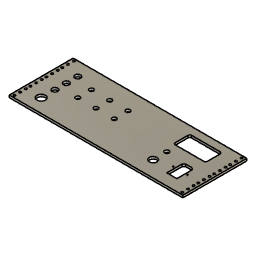
front_panel_3 v4 (Autodesk Fusion 360 design; units mm, degrees)
Autodesk Fusion 360 part; units mm, degrees
sketch "Sketch1" plane through (0, 0, 0) normal (0, 0, 1) x (1, 0, 0)
  line L0 (0, 0) -> (482.6, 0)
  line L1 (482.6, 0) -> (482.6, 177.8)
  line L2 (482.6, 177.8) -> (0, 177.8)
  line L3 (0, 177.8) -> (0, 0)
  dimension "d1" = 482.6
  dimension "d2" = 177.8
  constraint horizontal L0
  constraint vertical L1
  constraint horizontal L2
  constraint vertical L3
  constraint coincident L0.start L3.end
  measures "d1" distance of L0.start L0.end
  measures "d2" distance of L0.start L2.end
extrude "Extrude1" add sketch "Sketch1" along normal blind 6.35
sketch "Sketch2" plane through (0, 0, 6.35) normal (0, 0, 1) x (-1, 0, 0)
  line L0 (0, -177.8) -> (0, 0)
  line L1 (0, 0) -> (-482.6, 0)
  line L2 (-482.6, 0) -> (-482.6, -177.8)
  line L3 (-482.6, -177.8) -> (0, -177.8)
  circle A0 centre (-7.9375, -6.35) radius 3
  circle A1 centre (-7.9375, -22.225) radius 3
  circle A2 centre (-7.9375, -38.1) radius 3
  line L4 (-482.6, -88.9) -> (0, -88.9)
  line L5 (-241.3, -177.8) -> (-241.3, 0)
  line L6 (0, -44.45) -> (-482.6, -44.45)
  circle A3 centre (-7.9375, -50.8) radius 3
  circle A4 centre (-7.9375, -66.675) radius 3
  circle A5 centre (-7.9375, -82.55) radius 3
  circle A6 centre (-7.9375, -171.45) radius 3
  circle A7 centre (-7.9375, -155.575) radius 3
  circle A8 centre (-7.9375, -127) radius 3
  circle A9 centre (-7.9375, -111.125) radius 3
  circle A10 centre (-7.9375, -95.25) radius 3
  circle A11 centre (-7.9375, -139.7) radius 3
  circle A12 centre (-474.6625, -171.45) radius 3
  circle A13 centre (-474.6625, -155.575) radius 3
  circle A14 centre (-474.6625, -139.7) radius 3
  circle A15 centre (-474.6625, -127) radius 3
  circle A16 centre (-474.6625, -111.125) radius 3
  circle A17 centre (-474.6625, -95.25) radius 3
  circle A18 centre (-474.6625, -82.55) radius 3
  circle A19 centre (-474.6625, -66.675) radius 3
  circle A20 centre (-474.6625, -50.8) radius 3
  circle A21 centre (-474.6625, -38.1) radius 3
  circle A22 centre (-474.6625, -22.225) radius 3
  circle A23 centre (-474.6625, -6.35) radius 3
  point P0 (-7.3025, -3.751)
  dimension "d5" = 6
  dimension "d6" = 6
  dimension "d7" = 6
  dimension "d8" = 15.875
  dimension "d9" = 15.875
  dimension "d10" = 7.9375
  dimension "d11" = 6.35
  dimension "d12" = 44.45
  dimension "d15" = 31.75
  constraint midpoint L2 L4.start
  constraint midpoint L0 L4.end
  constraint midpoint L3 L5.start
  constraint midpoint L1 L5.end
  constraint coincident L0 L6.start
  constraint coincident L2 L6.end
  constraint perpendicular L2 L6
  constraint symmetric A0 L6 A5
  constraint symmetric A1 L6 A4
  constraint symmetric A2 L6 A3
  constraint symmetric A0 L4 A6
  constraint symmetric A1 L4 A7
  constraint symmetric A2 L4 A11
  constraint symmetric L4 A3 A8
  constraint symmetric L4 A4 A9
  constraint symmetric L4 A5 A10
  constraint symmetric A0 L5 A23
  constraint symmetric A1 L5 A22
  constraint symmetric A2 L5 A21
  constraint symmetric L5 A3 A20
  constraint symmetric L5 A4 A19
  constraint symmetric L5 A5 A18
  constraint symmetric L5 A6 A12
  constraint symmetric L5 A7 A13
  constraint symmetric L5 A8 A15
  constraint symmetric L5 A9 A16
  constraint symmetric L5 A10 A17
  constraint symmetric L5 A11 A14
  measures "d5" diameter of A0
  measures "d6" diameter of A2
  measures "d7" diameter of A1
  measures "d8" distance of A0.centre A1.centre
  measures "d9" distance of A2.centre A1.centre
  measures "d10" distance of L0 A0.centre
  measures "d11" distance of L1 A0.centre
  measures "d12" distance of L1 L6
  measures "d15" distance of A2.centre A0.centre
extrude "Extrude2" cut sketch "Sketch2" against normal blind 6.35 contours A0 | A1 | A2 | A3 | A4 | A5 | A6 | A7 | A8 | A9 | A10 | A11 | A12 | A13 | A14 | A15 | A16 | A17 | A18 | A19 | A20 | A21 | A22 | A23
sketch "Sketch3" plane through (0, 0, 6.35) normal (0, 0, 1) x (-1, 0, 0)
  circle A0 centre (-474.6625, -38.1) radius 3
  circle A1 centre (-474.6625, -171.45) radius 3
  circle A2 centre (-474.6625, -139.7) radius 3
  circle A3 centre (-7.9375, -38.1) radius 3
  circle A4 centre (-7.9375, -95.25) radius 3
  circle A5 centre (-7.9375, -155.575) radius 3
  circle A6 centre (-7.9375, -139.7) radius 3
  circle A7 centre (-7.9375, -82.55) radius 3
  circle A8 centre (-7.9375, -22.225) radius 3
  circle A9 centre (-474.6625, -127) radius 3
  circle A10 centre (-474.6625, -82.55) radius 3
  circle A11 centre (-474.6625, -22.225) radius 3
  circle A12 centre (-474.6625, -50.8) radius 3
  circle A13 centre (-474.6625, -95.25) radius 3
  circle A14 centre (-474.6625, -155.575) radius 3
  circle A15 centre (-7.9375, -50.8) radius 3
  circle A16 centre (-7.9375, -111.125) radius 3
  circle A17 centre (-7.9375, -171.45) radius 3
  circle A18 centre (-7.9375, -127) radius 3
  circle A19 centre (-7.9375, -66.675) radius 3
  circle A20 centre (-7.9375, -6.35) radius 3
  circle A21 centre (-474.6625, -111.125) radius 3
  circle A22 centre (-474.6625, -66.675) radius 3
  circle A23 centre (-474.6625, -6.35) radius 3
  line L0 (0, -177.8) -> (0, 0)
  line L1 (0, 0) -> (-482.6, 0)
  line L2 (-482.6, 0) -> (-482.6, -177.8)
  line L3 (-482.6, -177.8) -> (0, -177.8)
  circle A24 centre (-50.8, -38.1) radius 11.9062
  dimension "d16" = 23.8125
  dimension "d17" = 38.1
  dimension "d18" = 50.8
  measures "d16" diameter of A24
  measures "d17" distance of L1 A24.centre
  measures "d18" distance of L0 A24.centre
extrude "Extrude3" cut sketch "Sketch3" against normal blind 6.35 contours A24
sketch "Sketch5" plane through (0, 0, 6.35) normal (0, 0, 1) x (-1, 0, 0)
  circle A0 centre (-50.8, -38.1) radius 11.9062
  circle A1 centre (-474.6625, -38.1) radius 3
  circle A2 centre (-474.6625, -171.45) radius 3
  circle A3 centre (-474.6625, -139.7) radius 3
  circle A4 centre (-7.9375, -38.1) radius 3
  circle A5 centre (-7.9375, -95.25) radius 3
  circle A6 centre (-7.9375, -155.575) radius 3
  circle A7 centre (-7.9375, -139.7) radius 3
  circle A8 centre (-7.9375, -82.55) radius 3
  circle A9 centre (-7.9375, -22.225) radius 3
  circle A10 centre (-474.6625, -127) radius 3
  circle A11 centre (-474.6625, -82.55) radius 3
  circle A12 centre (-474.6625, -22.225) radius 3
  circle A13 centre (-474.6625, -50.8) radius 3
  circle A14 centre (-474.6625, -95.25) radius 3
  circle A15 centre (-474.6625, -155.575) radius 3
  circle A16 centre (-7.9375, -50.8) radius 3
  circle A17 centre (-7.9375, -111.125) radius 3
  circle A18 centre (-7.9375, -171.45) radius 3
  circle A19 centre (-7.9375, -127) radius 3
  circle A20 centre (-7.9375, -66.675) radius 3
  circle A21 centre (-7.9375, -6.35) radius 3
  circle A22 centre (-474.6625, -111.125) radius 3
  circle A23 centre (-474.6625, -66.675) radius 3
  circle A24 centre (-474.6625, -6.35) radius 3
  line L0 (0, -177.8) -> (0, 0)
  line L1 (0, 0) -> (-482.6, 0)
  line L2 (-482.6, 0) -> (-482.6, -177.8)
  line L3 (-482.6, -177.8) -> (0, -177.8)
  line L4 (-411.1625, -78.994) -> (-429.5775, -78.994)
  line L5 (-434.34, -31.75) -> (-406.4, -31.75)
  line L6 (-406.4, -31.75) -> (-406.4, -74.2315)
  line L7 (-429.5775, -78.994) -> (-434.34, -74.2315)
  circle A25 centre (-440.182, -55.372) radius 1.905
  line L8 (-434.34, -74.2315) -> (-434.34, -31.75)
  line L9 (-411.1625, -78.994) -> (-406.4, -74.2315)
  circle A26 centre (-400.558, -55.372) radius 1.905
  point P0 (-434.34, -78.994)
  point P1 (-406.4, -78.994)
  dimension "d32" = 27.94
  dimension "d33" = 47.244
  dimension "d34" = 3.81
  dimension "d35" = 3.81
  dimension "d36" = 23.622
  dimension "d37" = 23.622
  dimension "d38" = 5.842
  dimension "d39" = 5.842
  dimension "d40" = 4.7625
  dimension "d41" = 4.7625
  dimension "d42" = 4.7625
  dimension "d43" = 4.7625
  dimension "d44" = 406.4
  dimension "d45" = 31.75
  constraint horizontal L4
  constraint vertical L8
  constraint horizontal L5
  constraint vertical L6
  constraint coincident P1 L4
  constraint coincident P1 L6
  constraint coincident P0 L4
  constraint coincident P0 L8
  measures "d32" distance of P0 P1
  measures "d33" distance of P1 L5.end
  measures "d34" diameter of A25
  measures "d35" diameter of A26
  measures "d36" distance of A26.centre L5
  measures "d37" distance of A25.centre L5
  measures "d38" distance of A25.centre L8
  measures "d39" distance of A26.centre L6
  measures "d40" distance of P1 L4.start
  measures "d41" distance of P1 L6.end
  measures "d42" distance of P0 L4.end
  measures "d43" distance of P0 L7.end
  measures "d44" distance of L0 L6
  measures "d45" distance of L1 L5
extrude "Extrude5" cut sketch "Sketch5" against normal blind 6.35 contours L4 L5 L6 L7 L8 L9 | A25 | A26
sketch "Sketch6" plane through (0, 0, 6.35) normal (0, 0, 1) x (-1, 0, 0)
  line L0 (-406.4, -74.2315) -> (-411.1625, -78.994)
  line L1 (-411.1625, -78.994) -> (-429.5775, -78.994)
  line L2 (-429.5775, -78.994) -> (-434.34, -74.2315)
  line L3 (-434.34, -74.2315) -> (-434.34, -31.75)
  line L4 (-434.34, -31.75) -> (-406.4, -31.75)
  line L5 (-406.4, -31.75) -> (-406.4, -74.2315)
  circle A0 centre (-400.558, -55.372) radius 1.905
  circle A1 centre (-440.182, -55.372) radius 1.905
  circle A2 centre (-50.8, -38.1) radius 11.9062
  circle A3 centre (-474.6625, -38.1) radius 3
  circle A4 centre (-474.6625, -171.45) radius 3
  circle A5 centre (-474.6625, -139.7) radius 3
  circle A6 centre (-7.9375, -38.1) radius 3
  circle A7 centre (-7.9375, -95.25) radius 3
  circle A8 centre (-7.9375, -155.575) radius 3
  circle A9 centre (-7.9375, -139.7) radius 3
  circle A10 centre (-7.9375, -82.55) radius 3
  circle A11 centre (-7.9375, -22.225) radius 3
  circle A12 centre (-474.6625, -127) radius 3
  circle A13 centre (-474.6625, -82.55) radius 3
  circle A14 centre (-474.6625, -22.225) radius 3
  circle A15 centre (-474.6625, -50.8) radius 3
  circle A16 centre (-474.6625, -95.25) radius 3
  circle A17 centre (-474.6625, -155.575) radius 3
  circle A18 centre (-7.9375, -50.8) radius 3
  circle A19 centre (-7.9375, -111.125) radius 3
  circle A20 centre (-7.9375, -171.45) radius 3
  circle A21 centre (-7.9375, -127) radius 3
  circle A22 centre (-7.9375, -66.675) radius 3
  circle A23 centre (-7.9375, -6.35) radius 3
  circle A24 centre (-474.6625, -111.125) radius 3
  circle A25 centre (-474.6625, -66.675) radius 3
  circle A26 centre (-474.6625, -6.35) radius 3
  line L6 (0, -177.8) -> (0, 0)
  line L7 (0, 0) -> (-482.6, 0)
  line L8 (-482.6, 0) -> (-482.6, -177.8)
  line L9 (-482.6, -177.8) -> (0, -177.8)
  circle A27 centre (-355.6, -44.45) radius 10.795
  circle A28 centre (-355.6, -82.55) radius 6.35
  dimension "d48" = 21.59
  dimension "d49" = 355.6
  dimension "d50" = 44.45
  dimension "d64" = 12.7
  dimension "d65" = 38.1
  measures "d48" diameter of A27
  measures "d49" distance of L6 A27.centre
  measures "d50" distance of L7 A27.centre
  measures "d64" diameter of A28
  measures "d65" distance of A27.centre A28.centre
extrude "Extrude6" cut sketch "Sketch6" against normal blind 6.35 contours A27 | A28
sketch "Sketch7" plane through (0, 0, 6.35) normal (0, 0, 1) x (-1, 0, 0)
  circle A0 centre (-355.6, -44.45) radius 10.795
  line L0 (-406.4, -74.2315) -> (-411.1625, -78.994)
  line L1 (-411.1625, -78.994) -> (-429.5775, -78.994)
  line L2 (-429.5775, -78.994) -> (-434.34, -74.2315)
  line L3 (-434.34, -74.2315) -> (-434.34, -31.75)
  line L4 (-434.34, -31.75) -> (-406.4, -31.75)
  line L5 (-406.4, -31.75) -> (-406.4, -74.2315)
  circle A1 centre (-400.558, -55.372) radius 1.905
  circle A2 centre (-440.182, -55.372) radius 1.905
  circle A3 centre (-50.8, -38.1) radius 11.9062
  circle A4 centre (-474.6625, -38.1) radius 3
  circle A5 centre (-474.6625, -171.45) radius 3
  circle A6 centre (-474.6625, -139.7) radius 3
  circle A7 centre (-7.9375, -38.1) radius 3
  circle A8 centre (-7.9375, -95.25) radius 3
  circle A9 centre (-7.9375, -155.575) radius 3
  circle A10 centre (-7.9375, -139.7) radius 3
  circle A11 centre (-7.9375, -82.55) radius 3
  circle A12 centre (-7.9375, -22.225) radius 3
  circle A13 centre (-474.6625, -127) radius 3
  circle A14 centre (-474.6625, -82.55) radius 3
  circle A15 centre (-474.6625, -22.225) radius 3
  circle A16 centre (-474.6625, -50.8) radius 3
  circle A17 centre (-474.6625, -95.25) radius 3
  circle A18 centre (-474.6625, -155.575) radius 3
  circle A19 centre (-7.9375, -50.8) radius 3
  circle A20 centre (-7.9375, -111.125) radius 3
  circle A21 centre (-7.9375, -171.45) radius 3
  circle A22 centre (-7.9375, -127) radius 3
  circle A23 centre (-7.9375, -66.675) radius 3
  circle A24 centre (-7.9375, -6.35) radius 3
  circle A25 centre (-474.6625, -111.125) radius 3
  circle A26 centre (-474.6625, -66.675) radius 3
  circle A27 centre (-474.6625, -6.35) radius 3
  line L6 (0, -177.8) -> (0, 0)
  line L7 (0, 0) -> (-482.6, 0)
  line L8 (-482.6, 0) -> (-482.6, -177.8)
  line L9 (-482.6, -177.8) -> (0, -177.8)
  arc A28 (-345.44, -115.6652) -> (-350.2025, -110.9027) centre (-350.2025, -115.6652) ccw
  arc A29 (-350.2025, -156.3688) -> (-345.44, -151.6062) centre (-350.2025, -151.6062) ccw
  line L10 (-350.2025, -156.3688) -> (-430.3395, -156.3688)
  arc A30 (-435.102, -151.6062) -> (-430.3395, -156.3687) centre (-430.3395, -151.6062) ccw
  line L11 (-430.3395, -110.9027) -> (-350.2025, -110.9027)
  arc A31 (-430.3395, -110.9027) -> (-435.102, -115.6653) centre (-430.3395, -115.6653) ccw
  line L12 (-435.102, -151.6062) -> (-435.102, -115.6653)
  line L13 (-345.44, -115.6652) -> (-345.44, -151.6062)
  line L14 (-435.102, -133.35) -> (-345.44, -133.35)
  circle A32 centre (-355.6, -82.55) radius 6.35
  point P0 (-345.44, -110.9027)
  point P1 (-435.102, -110.9027)
  point P2 (-435.102, -156.3688)
  dimension "d53" = 89.662
  dimension "d54" = 45.466
  dimension "d55" = 23.0187
  dimension "d56" = 4.7625
  dimension "d57" = 4.7625
  dimension "d58" = 4.7625
  dimension "d59" = 4.7625
  dimension "d60" = 345.44
  dimension "d61" = 44.45
  constraint horizontal L11
  constraint vertical L13
  constraint horizontal L10
  constraint vertical L12
  constraint coincident L14.start L12
  constraint coincident L14.end L13
  constraint perpendicular L13 L14
  constraint coincident P1 L11
  constraint coincident P1 L12
  constraint tangent L11 A31
  constraint tangent A31 L12
  constraint coincident P0 L11
  constraint coincident P0 L13
  constraint tangent A28 L11
  constraint tangent A28 L13
  constraint tangent A29 L13
  constraint tangent A29 L10
  constraint coincident P2 L10
  constraint coincident P2 L12
  constraint tangent L10 A30
  constraint tangent A30 L12
  measures "d53" distance of P0 P1
  measures "d54" distance of P1 P2
  measures "d55" distance of L10 L14
  measures "d56" radius of A31
  measures "d57" radius of A28
  measures "d58" radius of A29
  measures "d59" radius of A30
  measures "d60" distance of L6 L13
  measures "d61" distance of L9 L14
extrude "Extrude7" cut sketch "Sketch7" against normal blind 6.35 contours A28 L11 A31 L12 L13 L14 | A29 L10 A30 L12 L13 L14
sketch "Sketch8" plane through (0, 0, 6.35) normal (0, 0, 1) x (-1, 0, 0)
  line L0 (-435.102, -151.6062) -> (-435.102, -115.6653)
  arc A0 (-430.3395, -110.9027) -> (-435.102, -115.6653) centre (-430.3395, -115.6653) ccw
  line L1 (-430.3395, -110.9027) -> (-350.2025, -110.9027)
  arc A1 (-345.44, -115.6652) -> (-350.2025, -110.9028) centre (-350.2025, -115.6652) ccw
  line L2 (-345.44, -115.6652) -> (-345.44, -151.6062)
  arc A2 (-350.2025, -156.3688) -> (-345.44, -151.6062) centre (-350.2025, -151.6063) ccw
  line L3 (-350.2025, -156.3688) -> (-430.3395, -156.3688)
  arc A3 (-435.102, -151.6063) -> (-430.3395, -156.3687) centre (-430.3395, -151.6062) ccw
  circle A4 centre (-355.6, -44.45) radius 10.795
  circle A5 centre (-355.6, -82.55) radius 6.35
  line L4 (-406.4, -74.2315) -> (-411.1625, -78.994)
  line L5 (-411.1625, -78.994) -> (-429.5775, -78.994)
  line L6 (-429.5775, -78.994) -> (-434.34, -74.2315)
  line L7 (-434.34, -74.2315) -> (-434.34, -31.75)
  line L8 (-434.34, -31.75) -> (-406.4, -31.75)
  line L9 (-406.4, -31.75) -> (-406.4, -74.2315)
  circle A6 centre (-400.558, -55.372) radius 1.905
  circle A7 centre (-440.182, -55.372) radius 1.905
  circle A8 centre (-50.8, -38.1) radius 11.9062
  circle A9 centre (-474.6625, -38.1) radius 3
  circle A10 centre (-474.6625, -171.45) radius 3
  circle A11 centre (-474.6625, -139.7) radius 3
  circle A12 centre (-7.9375, -38.1) radius 3
  circle A13 centre (-7.9375, -95.25) radius 3
  circle A14 centre (-7.9375, -155.575) radius 3
  circle A15 centre (-7.9375, -139.7) radius 3
  circle A16 centre (-7.9375, -82.55) radius 3
  circle A17 centre (-7.9375, -22.225) radius 3
  circle A18 centre (-474.6625, -127) radius 3
  circle A19 centre (-474.6625, -82.55) radius 3
  circle A20 centre (-474.6625, -22.225) radius 3
  circle A21 centre (-474.6625, -50.8) radius 3
  circle A22 centre (-474.6625, -95.25) radius 3
  circle A23 centre (-474.6625, -155.575) radius 3
  circle A24 centre (-7.9375, -50.8) radius 3
  circle A25 centre (-7.9375, -111.125) radius 3
  circle A26 centre (-7.9375, -171.45) radius 3
  circle A27 centre (-7.9375, -127) radius 3
  circle A28 centre (-7.9375, -66.675) radius 3
  circle A29 centre (-7.9375, -6.35) radius 3
  circle A30 centre (-474.6625, -111.125) radius 3
  circle A31 centre (-474.6625, -66.675) radius 3
  circle A32 centre (-474.6625, -6.35) radius 3
  line L10 (0, -177.8) -> (0, 0)
  line L11 (0, 0) -> (-482.6, 0)
  line L12 (-482.6, 0) -> (-482.6, -177.8)
  line L13 (-482.6, -177.8) -> (0, -177.8)
  circle A33 centre (-101.6, -88.9) radius 5.969
  circle A34 centre (-152.4, -88.9) radius 5.969
  circle A35 centre (-203.2, -88.9) radius 5.969
  circle A36 centre (-101.6, -127) radius 5.969
  circle A37 centre (-152.4, -127) radius 5.969
  circle A38 centre (-203.2, -127) radius 5.969
  dimension "d73" = 11.938
  dimension "d74" = 88.9
  dimension "d76" = 101.6
  dimension "d80" = -101.6
  dimension "d81" = -38.1
  measures "d73" diameter of A33
  measures "d74" distance of L11 A33.centre
  measures "d76" distance of L10 A33.centre
extrude "Extrude8" cut sketch "Sketch8" against normal blind 6.35 contours A33 | A34 | A35 | A36 | A37 | A38
sketch "Sketch9" plane through (0, 0, 6.35) normal (0, 0, 1) x (-1, 0, 0)
  circle A0 centre (-152.4, -127) radius 5.969
  circle A1 centre (-101.6, -127) radius 5.969
  circle A2 centre (-203.2, -127) radius 5.969
  circle A3 centre (-152.4, -88.9) radius 5.969
  circle A4 centre (-101.6, -88.9) radius 5.969
  circle A5 centre (-203.2, -88.9) radius 5.969
  line L0 (-435.102, -151.6062) -> (-435.102, -115.6653)
  arc A6 (-430.3395, -110.9027) -> (-435.102, -115.6653) centre (-430.3395, -115.6653) ccw
  line L1 (-430.3395, -110.9027) -> (-350.2025, -110.9027)
  arc A7 (-345.44, -115.6652) -> (-350.2025, -110.9028) centre (-350.2025, -115.6652) ccw
  line L2 (-345.44, -115.6652) -> (-345.44, -151.6062)
  arc A8 (-350.2025, -156.3688) -> (-345.44, -151.6062) centre (-350.2025, -151.6063) ccw
  line L3 (-350.2025, -156.3688) -> (-430.3395, -156.3688)
  arc A9 (-435.102, -151.6063) -> (-430.3395, -156.3687) centre (-430.3395, -151.6062) ccw
  circle A10 centre (-355.6, -44.45) radius 10.795
  circle A11 centre (-355.6, -82.55) radius 6.35
  line L4 (-406.4, -74.2315) -> (-411.1625, -78.994)
  line L5 (-411.1625, -78.994) -> (-429.5775, -78.994)
  line L6 (-429.5775, -78.994) -> (-434.34, -74.2315)
  line L7 (-434.34, -74.2315) -> (-434.34, -31.75)
  line L8 (-434.34, -31.75) -> (-406.4, -31.75)
  line L9 (-406.4, -31.75) -> (-406.4, -74.2315)
  circle A12 centre (-400.558, -55.372) radius 1.905
  circle A13 centre (-440.182, -55.372) radius 1.905
  circle A14 centre (-50.8, -38.1) radius 11.9062
  circle A15 centre (-474.6625, -38.1) radius 3
  circle A16 centre (-474.6625, -171.45) radius 3
  circle A17 centre (-474.6625, -139.7) radius 3
  circle A18 centre (-7.9375, -38.1) radius 3
  circle A19 centre (-7.9375, -95.25) radius 3
  circle A20 centre (-7.9375, -155.575) radius 3
  circle A21 centre (-7.9375, -139.7) radius 3
  circle A22 centre (-7.9375, -82.55) radius 3
  circle A23 centre (-7.9375, -22.225) radius 3
  circle A24 centre (-474.6625, -127) radius 3
  circle A25 centre (-474.6625, -82.55) radius 3
  circle A26 centre (-474.6625, -22.225) radius 3
  circle A27 centre (-474.6625, -50.8) radius 3
  circle A28 centre (-474.6625, -95.25) radius 3
  circle A29 centre (-474.6625, -155.575) radius 3
  circle A30 centre (-7.9375, -50.8) radius 3
  circle A31 centre (-7.9375, -111.125) radius 3
  circle A32 centre (-7.9375, -171.45) radius 3
  circle A33 centre (-7.9375, -127) radius 3
  circle A34 centre (-7.9375, -66.675) radius 3
  circle A35 centre (-7.9375, -6.35) radius 3
  circle A36 centre (-474.6625, -111.125) radius 3
  circle A37 centre (-474.6625, -66.675) radius 3
  circle A38 centre (-474.6625, -6.35) radius 3
  line L10 (0, -177.8) -> (0, 0)
  line L11 (0, 0) -> (-482.6, 0)
  line L12 (-482.6, 0) -> (-482.6, -177.8)
  line L13 (-482.6, -177.8) -> (0, -177.8)
  circle A39 centre (-50.8, -139.7) radius 8.001
  circle A40 centre (-50.8, -107.95) radius 8.001
  circle A41 centre (-50.8, -76.2) radius 8.001
  dimension "d84" = 16.002
  dimension "d87" = 0
  dimension "d88" = 63.5
  dimension "d89" = 38.1
  dimension "d90" = 50.8
  measures "d84" diameter of A39
  measures "d89" distance of L13 A39.centre
  measures "d90" distance of L10 A39.centre
extrude "Extrude9" cut sketch "Sketch9" against normal blind 6.35 contours A39 | A40 | A41
equation "d10 = ( 0.625 / 2 ) * 1 in"
